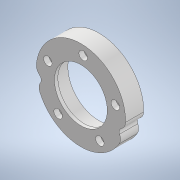
# Autodesk Inventor part: koszyczek
Saved by Autodesk Inventor 2022 (Build 260153000, 153)
## iProperties
Created: 2023-01-20
Part Number: koszyczek
Material: Generic
Document SubType Name: Modeling
Designer: Kamil
Density: 1 g/cm^3
Appearance: Default
Author: Kamil
Autodesk Inventor part; units mm, degrees
ref_plane "YZ Plane" through (0, 0, 0) normal (1, 0, 0) x (0, 1, 0)
ref_plane "XZ Plane" through (0, 0, 0) normal (0, 1, 0) x (-1, 0, 0)
ref_plane "XY Plane" through (0, 0, 0) normal (0, 0, 1) x (1, 0, 0)
sketch "Sketch1" plane through (0, 0, 0) normal (0, 0, 1) x (1, 0, 0)
  circle A0 centre (0, 0) radius 26.5 projected
  circle A1 centre (0, 0) radius 23.3333 projected
  circle A2 centre (0, 0) radius 27.5 projected
  circle A3 centre (0, 0) radius 19.1667 projected
  arc A4 (45.9013, -3.0114) -> (-45.9013, 3.0114) centre (0, 0) ccw projected
  line L0 (-45.9013, 3.0114) -> (-49.0763, -45.3846) projected
  line L1 (-49.0763, -45.3846) -> (360.9575, -72.2849) projected
  arc A5 (360.9575, -72.2849) -> (364.1325, -23.8889) centre (362.545, -48.0869) ccw projected
  line L2 (364.1325, -23.8889) -> (45.9013, -3.0114) projected
  circle A6 centre (-41.1996, -39.8885) radius 2 projected
  circle A7 centre (35.6352, -44.9292) radius 2 projected
  circle A8 centre (-38.9739, -5.9614) radius 2 projected
  circle A9 centre (37.861, -11.0021) radius 2 projected
  circle A10 centre (0, 0) radius 23.3333 projected
  line L3 (0, 27.5) -> (0, 39.5)
  line L4 (45.9013, -3.0114) -> (42.7263, -51.4073)
  line L5 (42.7263, -51.4073) -> (-49.0763, -45.3846)
  line L6 (-3.175, -48.396) -> (0, 0)
  line L7 (0, 0) -> (3.0114, 45.9013)
  line L8 (1.8003, 27.441) -> (2.5858, 39.4153)
  circle A11 centre (0, 0) radius 39.5
  line L9 (-1.8003, -27.441) -> (-2.5858, -39.4153)
  circle A12 centre (0, 33.5) radius 2
  circle A13 centre (-31.8604, 10.3521) radius 2
  circle A14 centre (-19.6908, -27.1021) radius 2
  circle A15 centre (19.6908, -27.1021) radius 2
  circle A16 centre (31.8604, 10.3521) radius 2
  circle A17 centre (-29.1794, 11.6435) radius 2.1 projected
  circle A18 centre (2.0567, 31.3493) radius 2.1 projected
  circle A19 centre (-20.0905, -24.1532) radius 2.1 projected
  circle A20 centre (30.4505, 7.7314) radius 2.1 projected
  circle A21 centre (16.7628, -26.571) radius 2.1 projected
  circle A22 centre (111.5584, -15.8371) radius 2 projected
  circle A23 centre (109.3326, -49.7641) radius 2 projected
  point P0 (0, 0)
  point P1 (-39.2982, -3.9879)
  point P2 (-38.6934, -7.9416)
  point P3 (37.3242, -12.9288)
  point P4 (38.4403, -9.0879)
  dimension "d0" = 12
  dimension "d1" = 12
  dimension "d2" = 4
  dimension "d5" = 360
  constraints: 14 end point, 6 centre point, 6 point on circle, 5 point on line, 2 midpoint, 2 perpendicular, 1 coincident, 1 collinear, 1 vertical, 11 other
  measures "d0" distance of L3.start L3.end
  measures "d1" distance of L8.start L8.end
  measures "d2" diameter of A12
extrude "Extrusion1" add sketch "Sketch1" along normal blind 3 contours A0 L6 A1 L7 | A0 L7 A2 L6 | L7 A1 L6 A0 | A0 L6 A2 L7 | L7 A18 A11 A9 L6 A2 | A2 L3 A18 L7 | L6 A11 A8 L3 A12 A18 A2 | A18 L3 A12 L7 | L7 A18 | A18 A12 L3 | A18 A12 L3 A11 L7 | A13 A17 | A14 A19 | A15 A21 | A16 A20 picked at (-0.0101, 31.1801) picked at (-28.183, 12.0138) picked at (-20.4544, -23.1407) picked at (15.6862, -26.6208) picked at (29.8267, 6.8653)
sketch "Sketch2" plane through (0, 0, 0) normal (0, 0, -1) x (-1, 0, 0)
  arc A0 (39.2982, -3.9879) -> (38.6934, -7.9416) centre (38.9739, -5.9614) ccw projected
  arc A1 (39.2982, -3.9879) -> (-38.4403, -9.0879) centre (0, 0) ccw projected
  arc A2 (-37.3242, -12.9288) -> (-38.4403, -9.0879) centre (-37.861, -11.0021) ccw projected
  arc A3 (-37.3242, -12.9288) -> (38.6934, -7.9416) centre (0, 0) ccw projected
  circle A4 centre (0, 0) radius 23.3333 projected
  circle A5 centre (0, 33.5) radius 2 projected
  circle A6 centre (-31.8604, 10.3521) radius 2 projected
  circle A7 centre (-19.6908, -27.1021) radius 2 projected
  circle A8 centre (31.8604, 10.3521) radius 2 projected
  circle A9 centre (19.6908, -27.1021) radius 2 projected
  point P0 (0, 0)
ref_plane "Work Plane1" through (-49.0763, -73.8724, -13) normal (0, 0, 1) x (0.9978549, -0.0654644, 0)
extrude "Extrusion2" add sketch "Sketch2" along normal up to surface (13 mm away)
sketch "Sketch3" plane through (0, 0, 3) normal (0, 0, 1) x (1, 0, 0)
  circle A0 centre (37.861, -11.0021) radius 2 projected
  arc A1 (-38.6934, -7.9416) -> (-39.2982, -3.9879) centre (-38.9739, -5.9614) ccw projected
  arc A2 (-38.6934, -7.9416) -> (37.3242, -12.9288) centre (0, 0) ccw projected
  arc A3 (38.4403, -9.0879) -> (37.3242, -12.9288) centre (37.861, -11.0021) ccw projected
  arc A4 (38.4403, -9.0879) -> (-39.2982, -3.9879) centre (0, 0) ccw projected
  circle A5 centre (0, 0) radius 23.3333 projected
  circle A6 centre (0, 33.5) radius 2 projected
  circle A7 centre (31.8604, 10.3521) radius 2 projected
  circle A8 centre (19.6908, -27.1021) radius 2 projected
  circle A9 centre (-31.8604, 10.3521) radius 2 projected
  circle A10 centre (-19.6908, -27.1021) radius 2 projected
  circle A11 centre (-38.9739, -5.9614) radius 2 projected
  circle A12 centre (-38.9739, -5.9614) radius 4
  circle A13 centre (37.861, -11.0021) radius 4
  point P0 (0, 0)
  dimension "d11" = 8
  dimension "d12" = 8
  constraints: 2 centre point, 2 coincident
  measures "d11" diameter of A12
  measures "d12" diameter of A13
extrude "Extrusion3" cut sketch "Sketch3" against normal through all contours A0 | A0 A4 A13 A2 | A0 A2 A13 A4 | A12 A2 A1 A4 | A4 A11 A2 A12 | A1 A11
fillet "Fillet1" radius 8 8 edges at (36.6205, -14.8049, 1.5) (36.6205, -14.8049, -6.5) (38.8518, -7.1268, 1.5) (38.8518, -7.1268, -6.5) (-38.2409, -9.8937, -6.5) (-38.2409, -9.8937, 1.5) (-39.4498, -1.9898, 1.5) (-39.4498, -1.9898, -6.5)
sketch "Sketch5" plane through (0, 0, -13) normal (0, 0, -1) x (-0.9978549, 0.0654644, 0)
  circle A0 centre (0, 0) radius 27.5 projected
  circle A1 centre (0, 0) radius 23.3333 projected
  point P0 (0, 0)
extrude "Extrusion5" cut sketch "Sketch5" against normal blind 13
sketch "Sketch6" plane through (0, 0, 3) normal (0, 0, 1) x (1, 0, 0)
  circle A0 centre (-19.6908, -27.1021) radius 2 projected
  circle A1 centre (-31.8604, 10.3521) radius 2 projected
  circle A2 centre (19.6908, -27.1021) radius 2 projected
  circle A3 centre (31.8604, 10.3521) radius 2 projected
  circle A4 centre (0, 33.5) radius 2 projected
  circle A5 centre (0, 0) radius 23.3333 projected
  arc A6 (-39.2843, 4.1223) -> (-36.4252, -2.8784) centre (-31.328, 3.2874) ccw projected
  arc A7 (-35.6202, -8.1415) -> (-36.4252, -2.8784) centre (-38.9739, -5.9614) ccw projected
  arc A8 (-35.6202, -8.1415) -> (-36.2558, -15.6768) centre (-28.9129, -12.5018) ccw projected
  arc A9 (-36.2558, -15.6768) -> (33.8969, -20.2792) centre (0, 0) ccw projected
  arc A10 (33.8969, -20.2792) -> (34.2512, -12.7254) centre (27.0317, -16.172) ccw projected
  arc A11 (35.737, -7.6127) -> (34.2512, -12.7254) centre (37.861, -11.0021) ccw projected
  arc A12 (35.737, -7.6127) -> (39.4862, -1.0454) centre (31.489, -0.8337) ccw projected
  arc A13 (39.4862, -1.0454) -> (-39.2843, 4.1223) centre (0, 0) ccw projected
  point P0 (0, 0)
ref_plane "Work Plane2" through (-49.0763, -73.8724, -13) normal (0, 0, 1) x (0.9978549, -0.0654644, 0)
extrude "Extrusion6" add sketch "Sketch6" against normal up to surface (16 mm away) contours A0 | A1 | A2 | A3 | A4
sketch "Sketch7" plane through (0, 0, 3) normal (0, 0, 1) x (1, 0, 0)
  arc A0 (45.9013, -3.0114) -> (-45.9013, 3.0114) centre (0, 0) ccw projected
  line L0 (-45.9013, 3.0114) -> (-49.0763, -45.3846) projected
  line L1 (-49.0763, -45.3846) -> (360.9575, -72.2849) projected
  arc A1 (360.9575, -72.2849) -> (364.1325, -23.8889) centre (362.545, -48.0869) ccw projected
  line L2 (364.1325, -23.8889) -> (45.9013, -3.0114) projected
  circle A2 centre (-41.1996, -39.8885) radius 2 projected
  circle A3 centre (35.6352, -44.9292) radius 2 projected
  circle A4 centre (-38.9739, -5.9614) radius 2 projected
  circle A5 centre (37.861, -11.0021) radius 2 projected
  circle A6 centre (0, 0) radius 23.3333 projected
  line L3 (0, 0) -> (-3.175, -48.396)
  line L4 (0, 0) -> (3.0114, 45.9013)
  arc A7 (39.4862, -1.0454) -> (-39.2843, 4.1223) centre (0, 0) ccw projected
  arc A8 (39.4862, -1.0454) -> (-39.2843, 4.1223) centre (0, 0) ccw projected
  line L5 (2.5858, 39.4153) -> (1.5275, 23.2833)
  circle A9 centre (0, 0) radius 23.3333 projected
  circle A10 centre (-29.1794, 11.6435) radius 2.1 projected
  circle A11 centre (2.0567, 31.3493) radius 2.1 projected
  circle A12 centre (-20.0905, -24.1532) radius 2.1 projected
  circle A13 centre (30.4505, 7.7314) radius 2.1 projected
  circle A14 centre (16.7628, -26.571) radius 2.1 projected
  circle A15 centre (111.5584, -15.8371) radius 2 projected
  circle A16 centre (109.3326, -49.7641) radius 2 projected
  point P0 (0, 0)
  point P1 (2.0567, 31.3493)
  point P2 (-29.1794, 11.6435)
  point P3 (-20.0905, -24.1532)
  point P4 (16.7628, -26.571)
  point P5 (30.4505, 7.7314)
  dimension "d29" = 360
  constraints: 6 end point, 2 point on circle, 2 point on line, 1 collinear, 1 midpoint, 1 perpendicular, 8 other
hole "Hole1" at (2.0567, 31.3493, 3) at (-29.1794, 11.6435, 3) at (-20.0905, -24.1532, 3) at (16.7628, -26.571, 3) at (30.4505, 7.7314, 3) direction (0, 0, -1) diameter 4.2 end through all counterbore diameter 7.5 counterbore depth 4.5
body "Solid1"
